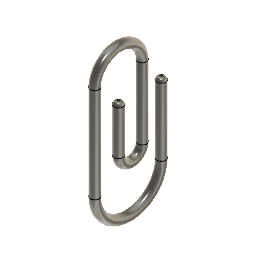
Semana2_Desafio5 (Autodesk Fusion 360 design; units mm, degrees)
Autodesk Fusion 360 part; units mm, degrees
note: some values were not read from the file. Chosen so that the rebuilt part matches the saved one: which face or edge a step refers to.
sketch "Sketch1" plane through (0, 0, 0) normal (0, 0, 1) x (1, 0, 0)
  circle A0 centre (0, 0) radius 1.9566
  constraint coincident A0.centre origin
sketch "Sketch2" plane through (0, 0, 0) normal (1, 0, 0) x (0, 1, 0)
  line L0 (0, 0) -> (0, 39.7926)
  arc A0 (20, 40) -> (0, 39.7926) centre (10.0011, 39.7926) ccw
  arc A1 (0, -0.0489) -> (28, 0) centre (14.0003, -0.1679) ccw
  line L1 (20, 40) -> (20, 10)
  arc A2 (10.0064, 10) -> (20, 10) centre (15.0032, 10) ccw
  line L2 (10.0064, 10) -> (10.0064, 30)
  line L3 (28, 0) -> (28, 30)
  constraint coincident L0.start origin
  constraint vertical L0
  constraint tangent L0 A0
  constraint vertical L1
  constraint tangent L1 A2
  constraint tangent A2 L2
  constraint parallel L1 L2
  constraint vertical L3
sketch "Sketch3" plane through (0, 0, 0) normal (0, 0, 1) x (1, 0, 0)
  circle A0 centre (0, 28) radius 1.9463
sweep "Sweep1" add profiles "Sketch1" path "Sketch2" along L0 A0 L1 A2 L2 section 1 makes body 1
sweep "Sweep2" add profiles "Sketch3" path "Sketch2" along A1 L3 section 1 separate body makes body 2
fillet "Fillet1" radius 1.5 1 faces at (-0.552, 9.8142, 30) on bodies 1
fillet "Fillet2" radius 1.5 1 edges at (-1.9463, 28, 30) on bodies 2
